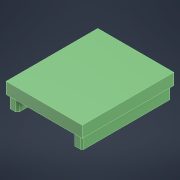
# Autodesk Inventor part: Logic_Level_Shifter
Saved by Autodesk Inventor 2022 (Build 260153000, 153)
## iProperties
Created: 2024-05-10
Part Number: Logic_Level_Shifter
Material: Generic
Document SubType Name: Modeling
Designer: jo_ki
Density: 1 g/cm^3
Appearance: Smooth - Dark Forest Green
Author: jo_ki
Autodesk Inventor part; units mm, degrees
ref_plane "YZ Plane" through (0, 0, 0) normal (1, 0, 0) x (0, 1, 0)
ref_plane "XZ Plane" through (0, 0, 0) normal (0, 1, 0) x (-1, 0, 0)
ref_plane "XY Plane" through (0, 0, 0) normal (0, 0, 1) x (1, 0, 0)
sketch "Sketch1" plane through (0, 0, 0) normal (0, 1, 0) x (-1, 0, 0)
  line L0 (-6.665, 8.025) -> (6.665, 8.025)
  line L1 (6.665, 8.025) -> (6.665, -8.025)
  line L2 (6.665, -8.025) -> (-6.665, -8.025)
  line L3 (-6.665, -8.025) -> (-6.665, 8.025)
  line L4 (-6.665, 8.025) -> (6.665, -8.025) construction
  line L5 (6.665, 8.025) -> (-6.665, -8.025) construction
  line L6 (0, -11.235) -> (0, 11.235) projected
  line L7 (6.665, 8.025) -> (4.665, 8.025)
  line L8 (4.665, 8.025) -> (4.665, -8.025)
  line L9 (4.665, -8.025) -> (6.665, -8.025)
  line L10 (6.665, -8.025) -> (6.665, 8.025)
  line L11 (-6.665, -8.025) -> (-4.665, -8.025)
  line L12 (-4.665, -8.025) -> (-4.665, 8.025)
  line L13 (-4.665, 8.025) -> (-6.665, 8.025)
  line L14 (-6.665, 8.025) -> (-6.665, -8.025)
  line L15 (4.865, -7.825) -> (4.865, 7.825)
  line L16 (4.865, 7.825) -> (6.465, 7.825)
  line L17 (6.465, 7.825) -> (6.465, -7.825)
  line L18 (6.465, -7.825) -> (4.865, -7.825)
  line L19 (-6.465, -7.825) -> (-4.865, -7.825)
  line L20 (-4.865, -7.825) -> (-4.865, 7.825)
  line L21 (-4.865, 7.825) -> (-6.465, 7.825)
  line L22 (-6.465, 7.825) -> (-6.465, -7.825)
  point P0 (0, 0)
  dimension "d0" = 16.05
  dimension "d1" = 13.33
  dimension "d7" = 2
  dimension "d8" = 0.2
  dimension "d9" = 0.2
  constraints: 44 end point, 10 parallel, 5 perpendicular, 3 horizontal, 2 midpoint, 2 point on line, 7 other
  measures "d0" distance of L0.end L1.end
  measures "d1" distance of L1.end L2.end
  measures "d7" distance between parallel lines of L1 L8
  measures "d8" distance between parallel lines of L8 L15
  measures "d9" distance between parallel lines of L14 L22
extrude "Extrusion1" add sketch "Sketch1" along normal blind 2 contours L0 L12 L2 L3 | L0 L6 L2 L12 | L0 L8 L2 L6 | L0 L1 L2 L8 | L15 L16 L17 L18 | L22 L21 L20 L19
extrude "Extrusion2" add sketch "Sketch1" against normal blind 2 contours L15 L16 L17 L18 | L22 L21 L20 L19
chamfer "Chamfer1" distance 0.3 angle 45 8 edges at (-4.865, -1, 7.825) (-6.465, -1, 7.825) (4.865, -1, 7.825) (6.465, -1, 7.825) (4.865, -1, -7.825) (6.465, -1, -7.825) (-4.865, -1, -7.825) (-6.465, -1, -7.825)
body "Solid1"
